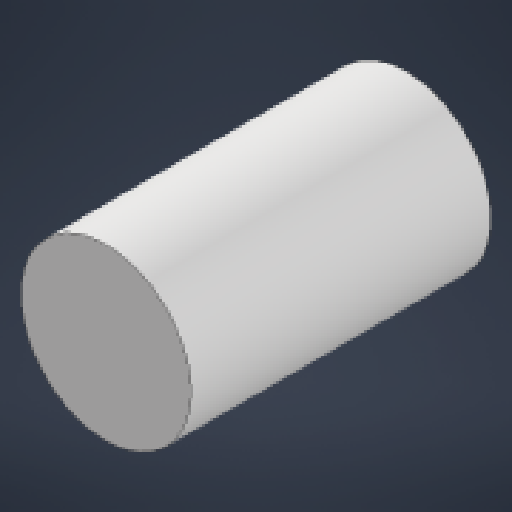
# Autodesk Inventor part: CarabinerThrowMount
Saved by Autodesk Inventor 2024.1 (Build 281209000, 209)
## iProperties
Created: 2023-10-16
Part Number: CarabinerThrowMount
Material: Generic
Document SubType Name: Modeling
Designer: Brandon
Density: 1 g/cm^3
Appearance: Default
Author: Brandon
Autodesk Inventor part; units mm, degrees
ref_plane "XZ Plane" through (0, 0, 0) normal (0, 1, 0) x (-1, 0, 0)
ref_plane "XY Plane" through (0, 0, 0) normal (0, 0, 1) x (1, 0, 0)
sketch "Sketch1" plane through (0, 0, 0) normal (0, 0, 1) x (1, 0, 0)
  line L0 (285.1848, -19.0386) -> (-264.1554, -38.0771) projected
  arc A0 (285.1848, -19.0386) -> (285.1848, 19.0386) centre (284.525, 0) ccw projected
  line L1 (-264.1554, 38.0771) -> (285.1848, 19.0386) projected
  arc A1 (-264.1554, 38.0771) -> (-264.1554, -38.0771) centre (-265.475, 0) ccw projected
  circle A2 centre (284.525, -9.525) radius 2 projected
  circle A3 centre (294.05, 0) radius 2 projected
  circle A4 centre (284.525, 9.525) radius 2 projected
  circle A5 centre (-290.875, 0) radius 2.1 projected
  circle A6 centre (-278.175, -21.997) radius 2.1 projected
  circle A7 centre (-252.775, -21.997) radius 2.1 projected
  circle A8 centre (-278.175, 21.997) radius 2.1 projected
  circle A9 centre (-252.775, 21.997) radius 2.1 projected
  line L2 (-252.775, -12.7) -> (-252.775, 12.7) projected
  line L3 (-278.175, -12.7) -> (-252.775, -12.7) projected
  line L4 (-278.175, 12.7) -> (-278.175, -12.7) projected
  line L5 (-252.775, 12.7) -> (-278.175, 12.7) projected
  circle A10 centre (-240.075, 0) radius 2.1 projected
  circle A11 centre (275, 0) radius 2 projected
  circle A12 centre (284.525, 0) radius 19.05
  circle A13 centre (275, 0) radius 2.7813
  circle A14 centre (284.525, 9.525) radius 2.7813
  circle A15 centre (294.05, 0) radius 2.7813
  circle A16 centre (284.525, -9.525) radius 2.7813
  point P0 (0, 0)
  dimension "d0" = 5.5626
  dimension "d1" = 5.5626
  dimension "d2" = 5.5626
  dimension "d3" = 5.5626
  constraints: 5 coincident, 4 centre point, 3 other
  measures "d0" diameter of A13
  measures "d1" diameter of A14
  measures "d2" diameter of A15
  measures "d3" diameter of A16
extrude "Extrusion1" add sketch "Sketch1" along normal blind 67.3 contours A12 A0 | A2 | A3 | A4 | A11 | A13 | A14 | A15 | A16
extrude "Extrusion2" cut sketch "Sketch1" along normal blind 8 contours A2 | A3 | A4 | A11 | A13 | A14 | A15 | A16
extrude "Extrusion3" cut sketch "Sketch1" along normal blind 19.05 contours A2 | A3 | A4 | A11
ref_plane "Work Plane1" through (284.525, 0, 33.65) normal (0, 0, -1) x (-1, 0, 0)
mirror "Mirror1" about plane through (284.525, 0, 33.65) normal (0, 0, -1) of "Extrusion2", "Extrusion3"
chamfer "Chamfer1" distance 0.635 angle 45 16 edges at (272.2187, 0, 67.3) (281.7437, 9.525, 67.3) (281.7437, -9.525, 67.3) (291.2687, 0, 67.3) (273, 0, 59.3) (282.525, -9.525, 59.3) (282.525, 9.525, 59.3) (292.05, 0, 59.3) (281.7437, 9.525, 0) (272.2187, 0, 0) (291.2687, 0, 0) (281.7437, -9.525, 0) (292.05, 0, 8) (282.525, -9.525, 8) (273, 0, 8) (282.525, 9.525, 8)
ref_plane "Work Plane3" through (284.525, 0, 0) normal (1, 0, 0) x (0, 1, 0)
sketch "Sketch3" plane through (284.525, 0, 0) normal (1, 0, 0) x (0, 1, 0)
  line L0 (19.05, 67.3) -> (-19.05, 67.3) projected
  line L1 (19.05, 0) -> (-19.05, 0) projected
  circle A0 centre (-19.05, 60.95) radius 6.35
  circle A1 centre (-19.05, 6.35) radius 6.35
  circle A2 centre (-19.05, 60.95) radius 3.81
  circle A3 centre (-19.05, 6.35) radius 3.81
  point P0 (0, 0)
  dimension "d15" = 12.7
  dimension "d16" = 12.7
  dimension "d17" = 7.62
  dimension "d18" = 7.62
  constraints: 2 centre point, 2 coincident, 2 horizontal, 2 vertical alignment, 4 other
  measures "d17" diameter of A2
  measures "d18" diameter of A3
extrude "Extrusion4" cut sketch "Sketch3" along normal through all both and the other way through all contours A2 | A3
extrude "Extrusion5" add sketch "Sketch3" along normal mid plane 5.08
chamfer "Chamfer2" distance 3.81 angle 45 8 edges at (287.065, -18.8799, 66.027) (287.065, -18.8799, 55.873) (287.065, -18.8799, 11.427) (287.065, -18.8799, 1.273) (281.985, -18.8799, 11.427) (281.985, -18.8799, 1.273) (281.985, -18.8799, 66.027) (281.985, -18.8799, 55.873)
body "Solid1"
